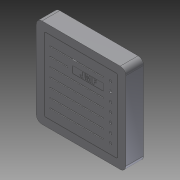
# Autodesk Inventor part: readerCase
Saved by Autodesk Inventor 2012 (Build 160160000, 160)
## iProperties
Created: 2013-12-15
Part Number: readerCase
Material: Default
Document SubType Name: Modeling
Designer: joe_000
Density: 1 g/cm^3
Author: joe_000
Autodesk Inventor part; units mm, degrees
ref_plane "YZ Plane" through (0, 0, 0) normal (1, 0, 0) x (0, 1, 0)
ref_plane "XZ Plane" through (0, 0, 0) normal (0, 1, 0) x (-1, 0, 0)
sketch "Sketch1" plane through (0, 0, 0) normal (0, 0, 1) x (1, 0, 0)
  line L0 (7.9375, 0) -> (119.0625, 0)
  line L1 (127, 7.9375) -> (127, 119.0625)
  line L2 (119.0625, 127) -> (7.9375, 127)
  line L3 (0, 119.0625) -> (0, 7.9375)
  arc A0 (119.0625, 0) -> (127, 7.9375) centre (119.0625, 7.9375) ccw
  arc A1 (127, 119.0625) -> (119.0625, 127) centre (119.0625, 119.0625) ccw
  arc A2 (7.9375, 127) -> (0, 119.0625) centre (7.9375, 119.0625) ccw
  arc A3 (0, 7.9375) -> (7.9375, 0) centre (7.9375, 7.9375) ccw
  point P0 (0, 0)
  point P1 (127, 0)
  point P2 (0, 127)
  dimension "d0" = 127
  dimension "d1" = 127
  dimension "d2" = 7.9375
  constraints: 8 end point, 8 point on circle, 8 tangent, 6 point on line, 4 centre point, 3 equal radius, 2 parallel, 1 horizontal, 1 perpendicular
  measures "d0" distance of point (0, 0) point (127, 0)
  measures "d1" distance of point (0, 127) point (0, 0)
  measures "d2" radius of A0
extrude "Extrusion1" add sketch "Sketch1" along normal blind 25.4
sketch "Sketch2" plane through (0, 0, 0) normal (0, 0, -1) x (-1, 0, 0)
  line L0 (-119.0625, 0) -> (-7.9375, 0) projected
  line L1 (0, 7.9375) -> (0, 119.0625) projected
  line L2 (-7.9375, 127) -> (-119.0625, 127) projected
  line L3 (-127, 119.0625) -> (-127, 7.9375) projected
  arc A0 (-127, 7.9375) -> (-119.0625, 0) centre (-119.0625, 7.9375) ccw projected
  line L4 (-119.0625, 125.4125) -> (-7.9375, 125.4125)
  line L5 (-1.5875, 119.0625) -> (-1.5875, 7.9375)
  line L6 (-7.9375, 1.5875) -> (-119.0625, 1.5875)
  line L7 (-125.4125, 7.9375) -> (-125.4125, 119.0625)
  arc A1 (-125.4125, 7.9375) -> (-119.0625, 1.5875) centre (-119.0625, 7.9375) ccw
  arc A2 (-119.0625, 125.4125) -> (-125.4125, 119.0625) centre (-119.0625, 119.0625) ccw
  arc A3 (-1.5875, 119.0625) -> (-7.9375, 125.4125) centre (-7.9375, 119.0625) ccw
  arc A4 (-7.9375, 1.5875) -> (-1.5875, 7.9375) centre (-7.9375, 7.9375) ccw
  point P0 (0, 0)
  dimension "d6" = 1.5875
  dimension "d7" = 1.5875
  dimension "d8" = 1.5875
  dimension "d9" = 1.5875
  dimension "d10" = 1.5875
  constraints: 8 end point, 8 point on circle, 8 tangent, 4 centre point, 3 equal radius, 2 parallel, 1 horizontal, 1 perpendicular
  measures "d6" distance between parallel lines of L3 L7
  measures "d7" distance between parallel lines of L2 L4
  measures "d8" distance between parallel lines of L1 L5
  measures "d9" distance between parallel lines of L0 L6
  measures "d10" radial gap between concentric circles of A0 A1
extrude "Extrusion2" cut sketch "Sketch2" against normal blind 23.8125
sketch "Sketch3" plane through (0, 0, 25.4) normal (0, 0, 1) x (1, 0, 0)
  line L0 (7.9375, 127) -> (119.0625, 127) projected
  line L1 (0, 7.9375) -> (0, 119.0625) projected
  line L2 (13.208, 115.824) -> (113.792, 115.824)
  line L3 (115.824, 113.792) -> (115.824, 13.208)
  line L4 (113.792, 11.176) -> (13.208, 11.176)
  line L5 (11.176, 13.208) -> (11.176, 113.792)
  line L6 (13.208, 115.4271) -> (113.792, 115.4271)
  line L7 (115.4271, 113.792) -> (115.4271, 13.208)
  line L8 (113.792, 11.5729) -> (13.208, 11.5729)
  line L9 (11.5729, 13.208) -> (11.5729, 113.792)
  arc A0 (13.208, 115.824) -> (11.176, 113.792) centre (13.208, 113.792) ccw
  arc A1 (11.176, 13.208) -> (13.208, 11.176) centre (13.208, 13.208) ccw
  arc A2 (113.792, 11.176) -> (115.824, 13.208) centre (113.792, 13.208) ccw
  arc A3 (115.824, 113.792) -> (113.792, 115.824) centre (113.792, 113.792) ccw
  arc A4 (13.208, 115.4271) -> (11.5729, 113.792) centre (13.208, 113.792) ccw
  arc A5 (115.4271, 113.792) -> (113.792, 115.4271) centre (113.792, 113.792) ccw
  arc A6 (113.792, 11.5729) -> (115.4271, 13.208) centre (113.792, 13.208) ccw
  arc A7 (11.5729, 13.208) -> (13.208, 11.5729) centre (13.208, 13.208) ccw
  point P0 (0, 0)
  dimension "d15" = 104.648
  dimension "d16" = 104.648
  dimension "d17" = 0.3969
  dimension "d18" = 0.3969
  dimension "d19" = 0.3969
  dimension "d20" = 0.3969
  dimension "d21" = 0.3969
  dimension "d22" = 11.176
  dimension "d23" = 11.176
  dimension "d24" = 2.032
  constraints: 16 end point, 16 point on circle, 16 tangent, 8 centre point, 6 equal radius, 4 parallel, 2 horizontal, 2 perpendicular
  measures "d15" distance between parallel lines of L4 L2
  measures "d16" distance between parallel lines of L3 L5
  measures "d17" distance between parallel lines of L2 L6
  measures "d18" distance between parallel lines of L3 L7
  measures "d19" distance between parallel lines of L4 L8
  measures "d20" distance between parallel lines of L5 L9
  measures "d21" radial gap between concentric circles of A0 A4
  measures "d22" distance between parallel lines of L1 L5
  measures "d23" distance between parallel lines of L0 L2
  measures "d24" radius of A0
extrude "Extrusion3" cut sketch "Sketch3" against normal blind 0.7937
sketch "Sketch4" plane through (0, 0, 25.4) normal (0, 0, 1) x (1, 0, 0)
  line L0 (119.0625, 0) -> (7.9375, 0) projected
  line L1 (127, 119.0625) -> (127, 7.9375) projected
  line L2 (0, 7.9375) -> (0, 119.0625) projected
  line L3 (19.304, 26.035) -> (95.504, 26.035)
  line L4 (95.504, 26.035) -> (95.504, 24.765)
  line L5 (95.504, 24.765) -> (19.304, 24.765)
  line L6 (19.304, 24.765) -> (19.304, 26.035)
  line L7 (19.304, 38.735) -> (95.504, 38.735)
  line L8 (95.504, 38.735) -> (95.504, 37.465)
  line L9 (95.504, 37.465) -> (19.304, 37.465)
  line L10 (19.304, 37.465) -> (19.304, 38.735)
  line L11 (19.304, 51.435) -> (95.504, 51.435)
  line L12 (95.504, 51.435) -> (95.504, 50.165)
  line L13 (95.504, 50.165) -> (19.304, 50.165)
  line L14 (19.304, 50.165) -> (19.304, 51.435)
  line L15 (19.304, 64.135) -> (95.504, 64.135)
  line L16 (95.504, 64.135) -> (95.504, 62.865)
  line L17 (95.504, 62.865) -> (19.304, 62.865)
  line L18 (19.304, 62.865) -> (19.304, 64.135)
  line L19 (19.304, 76.835) -> (95.504, 76.835)
  line L20 (95.504, 76.835) -> (95.504, 75.565)
  line L21 (95.504, 75.565) -> (19.304, 75.565)
  line L22 (19.304, 75.565) -> (19.304, 76.835)
  line L23 (19.304, 102.235) -> (95.504, 102.235)
  line L24 (95.504, 102.235) -> (95.504, 100.965)
  line L25 (95.504, 100.965) -> (19.304, 100.965)
  line L26 (19.304, 100.965) -> (19.304, 102.235)
  line L27 (19.304, 89.535) -> (44.704, 89.535)
  line L28 (44.704, 89.535) -> (44.704, 88.265)
  line L29 (44.704, 88.265) -> (19.304, 88.265)
  line L30 (19.304, 88.265) -> (19.304, 89.535)
  point P0 (0, 0)
  dimension "d27" = 24.765
  dimension "d28" = 1.27
  dimension "d29" = 19.304
  dimension "d30" = 76.2
  dimension "d33" = 12.7
  dimension "d40" = 76.2
  dimension "d45" = 25.4
  dimension "d46" = 12.7
  constraints: 56 end point, 4 parallel, 2 collinear, 2 horizontal, 2 perpendicular, 2 vertical, 40 other
  measures "d27" distance between parallel lines of L0 L5
  measures "d28" distance of L5.end L3.start
  measures "d29" distance between parallel lines of L2 L6
  measures "d30" distance of L4.end L5.end
  measures "d33" distance of L3.start L10.end
  measures "d40" distance of L3.end L23.end
  measures "d45" distance of L27.start L27.end
  measures "d46" distance from line of L29 L22.start
extrude "Extrusion4" cut sketch "Sketch4" against normal blind 0.7937
sketch "Sketch6" plane through (0, 0, 25.4) normal (0, 0, 1) x (1, 0, 0)
  line L0 (119.0625, 0) -> (7.9375, 0) projected
  line L1 (127, 119.0625) -> (127, 7.9375) projected
  circle A0 centre (105.41, 25.4) radius 1.905
  circle A1 centre (105.41, 38.1) radius 1.905
  circle A2 centre (105.41, 50.8) radius 1.905
  circle A3 centre (105.41, 63.5) radius 1.905
  circle A4 centre (105.41, 76.2) radius 1.905
  circle A5 centre (105.41, 88.9) radius 1.905
  circle A6 centre (105.41, 101.6) radius 1.905
  point P0 (0, 0)
  dimension "d53" = 3.81
  dimension "d56" = 12.7
  dimension "d61" = 21.59
  dimension "d62" = 25.4
  constraints: 7 centre point, 1 vertical, 12 other
  measures "d53" diameter of A0
  measures "d56" distance of A0.centre A1.centre
  measures "d61" distance from line of L1 A0.centre
  measures "d62" distance from line of L0 A0.centre
extrude "Extrusion6" cut sketch "Sketch6" against normal blind 0.7937
sketch "Sketch7" plane through (0, 0, 25.4) normal (0, 0, 1) x (1, 0, 0)
  circle A0 centre (105.41, 88.9) radius 1.905 projected
  circle A1 centre (105.41, 88.9) radius 1.905
  point P0 (0, 0)
  constraints: 1 centre point, 1 coincident, 1 concentric
extrude "Extrusion7" cut sketch "Sketch7" against normal up to next
sketch "Sketch5" plane through (0, 0, 25.4) normal (0, 0, 1) x (1, 0, 0)
  line L0 (19.304, 100.965) -> (19.304, 102.235) projected
  line L1 (19.304, 102.235) -> (95.504, 102.235) projected
  line L2 (95.504, 100.965) -> (19.304, 100.965) projected
  line L3 (51.054, 102.235) -> (56.134, 102.235)
  line L4 (56.134, 102.235) -> (56.134, 100.965)
  line L5 (56.134, 100.965) -> (51.054, 100.965)
  line L6 (51.054, 100.965) -> (51.054, 102.235)
  point P0 (0, 0)
  dimension "d49" = 5.08
  dimension "d50" = 31.75
  constraints: 8 end point, 2 parallel, 2 point on line, 1 horizontal, 1 perpendicular
  measures "d49" distance of L3.start L3.end
  measures "d50" distance between parallel lines of L0 L6
extrude "Extrusion5" cut sketch "Sketch5" against normal up to next contours L6 L1 L4 L2
sketch "Sketch8" plane through (0, 0, 25.4) normal (0, 0, 1) x (1, 0, 0)
  line L0 (7.9375, 127) -> (119.0625, 127) projected
  line L1 (52.324, 93.98) -> (94.234, 93.98)
  line L2 (95.504, 92.71) -> (95.504, 85.344)
  line L3 (94.234, 84.074) -> (52.324, 84.074)
  line L4 (51.054, 85.344) -> (51.054, 92.71)
  arc A0 (52.324, 93.98) -> (51.054, 92.71) centre (52.324, 92.71) ccw
  arc A1 (51.054, 85.344) -> (52.324, 84.074) centre (52.324, 85.344) ccw
  arc A2 (95.504, 92.71) -> (94.234, 93.98) centre (94.234, 92.71) ccw
  arc A3 (94.234, 84.074) -> (95.504, 85.344) centre (94.234, 85.344) ccw
  line L5 (95.504, 102.235) -> (95.504, 100.965) projected
  point P0 (0, 0)
  dimension "d67" = 1.27
  dimension "d68" = 9.906
  dimension "d69" = 44.45
  dimension "d70" = 33.02
  constraints: 8 end point, 8 point on circle, 8 tangent, 4 centre point, 3 equal radius, 2 parallel, 1 collinear, 1 horizontal, 1 perpendicular
  measures "d67" radius of A0
  measures "d68" distance between parallel lines of L3 L1
  measures "d69" distance between parallel lines of L2 L4
  measures "d70" distance between parallel lines of L0 L1
extrude "Extrusion8" cut sketch "Sketch8" against normal blind 0.3969
sketch "Sketch9" plane through (0, 0, 25.4) normal (0, 0, 1) x (1, 0, 0)
  line L0 (52.324, 93.98) -> (94.234, 93.98) projected
  line L1 (51.054, 85.344) -> (51.054, 92.71) projected
  line L2 (61.214, 92.837) -> (85.344, 92.837) construction
  line L3 (85.344, 92.837) -> (85.344, 85.217) construction
  line L4 (85.344, 85.217) -> (61.214, 85.217) construction
  line L5 (61.214, 85.217) -> (61.214, 92.837) construction
  line L6 (65.1597, 92.837) -> (67.5212, 92.837)
  line L7 (67.5212, 92.837) -> (67.5212, 88.6933)
  spline S0 degree 2 poles (67.5212, 88.6933) (67.5212, 87.3952) (67.0592, 86.0311) (65.6584, 85.085) (64.573, 85.085) knots 0 0 0 1 2 3 3 3
  spline S1 degree 2 poles (64.573, 85.085) (63.4215, 85.085) (62.1527, 85.7084) (61.4634, 86.9111) (61.3973, 87.7912) knots 0 0 0 1 2 3 3 3
  line L8 (61.3973, 87.7912) -> (63.6489, 88.0993)
  spline S2 degree 2 poles (63.6489, 88.0993) (63.6562, 87.5932) (63.8176, 87.1092) (64.0156, 86.9552) knots 0 0 0 1 2 2 2
  spline S3 degree 2 poles (64.0156, 86.9552) (64.1476, 86.8598) (64.3969, 86.8598) knots 0 0 0 1 1 1
  spline S4 degree 2 poles (64.3969, 86.8598) (64.793, 86.8598) (65.1597, 87.4465) (65.1597, 88.1433) knots 0 0 0 1 2 2 2
  line L9 (65.1597, 88.1433) -> (65.1597, 92.837)
  line L10 (69.076, 92.837) -> (72.1783, 92.837)
  line L11 (72.1783, 92.837) -> (73.3664, 88.2019)
  line L12 (73.3664, 88.2019) -> (74.5472, 92.837)
  line L13 (74.5472, 92.837) -> (77.6421, 92.837)
  line L14 (77.6421, 92.837) -> (77.6421, 85.217)
  line L15 (77.6421, 85.217) -> (75.7133, 85.217)
  line L16 (75.7133, 85.217) -> (75.7133, 91.0328)
  line L17 (75.7133, 91.0328) -> (74.2318, 85.217)
  line L18 (74.2318, 85.217) -> (72.4863, 85.217)
  line L19 (72.4863, 85.217) -> (71.0049, 91.0328)
  line L20 (71.0049, 91.0328) -> (71.0049, 85.217)
  line L21 (71.0049, 85.217) -> (69.076, 85.217)
  line L22 (69.076, 85.217) -> (69.076, 92.837)
  line L23 (79.1676, 92.837) -> (84.9834, 92.837)
  line L24 (84.9834, 92.837) -> (84.9834, 91.2015)
  line L25 (84.9834, 91.2015) -> (81.5364, 91.2015)
  line L26 (81.5364, 91.2015) -> (81.5364, 89.8741)
  line L27 (81.5364, 89.8741) -> (84.4774, 89.8741)
  line L28 (84.4774, 89.8741) -> (84.4774, 88.3339)
  line L29 (84.4774, 88.3339) -> (81.5364, 88.3339)
  line L30 (81.5364, 88.3339) -> (81.5364, 85.217)
  line L31 (81.5364, 85.217) -> (79.1676, 85.217)
  line L32 (79.1676, 85.217) -> (79.1676, 92.837)
  point P0 (0, 0)
  dimension "d74" = 1.143
  dimension "d75" = 10.16
  dimension "d76" = 24.13
  constraints: 2 other
  measures "d74" distance between parallel lines of L0 L2
  measures "d75" distance between parallel lines of L1 L5
  measures "d76" distance between parallel lines of L3 L5
extrude "Extrusion9" cut sketch "Sketch9" against normal blind 0.7937
sketch "Sketch10" plane through (0, 0, 23.8125) normal (0, 0, -1) x (-1, 0, 0)
  line L0 (-1.5875, 7.9375) -> (-1.5875, 119.0625) projected
  line L1 (-33.7625, 118.1275) -> (-1.5875, 118.1275)
  line L2 (-1.5875, 118.1275) -> (-1.5875, 8.8725)
  line L3 (-1.5875, 8.8725) -> (-33.7625, 8.8725)
  line L4 (-33.7625, 8.8725) -> (-33.7625, 118.1275)
  line L5 (-119.0625, 0) -> (-7.9375, 0) projected
  point P0 (0, 0)
  dimension "d79" = 109.255
  dimension "d80" = 8.8725
  dimension "d81" = 32.175
  constraints: 8 end point, 2 parallel, 1 horizontal, 1 perpendicular, 1 point on line
  measures "d79" distance of L3.end L1.start
  measures "d80" distance between parallel lines of L5 L3
  measures "d81" distance between parallel lines of L2 L4
extrude "Extrusion10" add sketch "Sketch10" along normal blind 16.0875
ref_plane "Work Plane2" through (1.5875, 10.46, 23.8125) normal (0, -1, 0) x (1, 0, 0)
sketch "Sketch12" plane through (1.5875, 10.46, 23.8125) normal (0, -1, 0) x (1, 0, 0)
  line L0 (0, -18.5759) -> (32.175, -18.5759)
  line L1 (32.175, 0) -> (32.175, -18.5759)
  line L2 (0, -18.5759) -> (0, 0)
  line L3 (1.5875, -18.5759) -> (1.5875, -8.7762)
  line L4 (30.5875, -18.5759) -> (30.5875, -8.7762)
  arc A0 (16.0875, -8.7762) -> (1.5875, -8.7762) centre (8.8375, -8.7762) ccw
  arc A1 (30.5875, -8.7762) -> (16.0875, -8.7762) centre (23.3375, -8.7762) ccw
  point P0 (-1.5875, -23.8125)
  dimension "d85" = 7.25
  dimension "d86" = 7.25
  dimension "d87" = 1.5875
  dimension "d88" = 1.5875
  constraints: 10 end point, 4 point on circle, 2 centre point, 2 horizontal alignment, 2 parallel, 2 point on line
  measures "d85" radius of A0
  measures "d86" radius of A1
  measures "d87" distance between parallel lines of L3 L2
  measures "d88" distance between parallel lines of L1 L4
extrude "Extrusion11" cut sketch "Sketch12" against normal blind 106.08
sketch "Sketch13" plane through (0, 0, 23.8125) normal (0, 0, -1) x (-1, 0, 0)
  line L0 (-125.4125, 119.0625) -> (-125.4125, 7.9375) projected
  line L1 (-119.0625, 1.5875) -> (-7.9375, 1.5875) projected
  circle A0 centre (-112.7125, 14.2875) radius 3.5
  circle A1 centre (-112.7125, 14.2875) radius 1.5
  circle A2 centre (-74.6125, 14.2875) radius 3.5
  circle A3 centre (-74.6125, 14.2875) radius 1.5
  circle A4 centre (-112.7125, 96.8375) radius 3.5
  circle A5 centre (-112.7125, 96.8375) radius 1.5
  circle A6 centre (-74.6125, 96.8375) radius 3.5
  circle A7 centre (-74.6125, 96.8375) radius 1.5
  point P0 (0, 0)
  dimension "d92" = 7
  dimension "d93" = 3
  dimension "d96" = 38.1
  dimension "d99" = 82.55
  dimension "d104" = 12.7
  dimension "d105" = 12.7
  constraints: 8 centre point, 4 coincident, 1 horizontal, 1 vertical, 12 other
  measures "d92" diameter of A0
  measures "d93" diameter of A1
  measures "d96" distance of A0.centre A2.centre
  measures "d99" distance of A0.centre A4.centre
  measures "d104" distance from line of L1 A1.centre
  measures "d105" distance from line of L0 A0.centre
extrude "Extrusion12" add sketch "Sketch13" along normal blind 10.38
equation "\"d7\" = d6"
equation "\"d8\" = d6"
equation "\"d9\" = d6"
equation "\"d10\" = d6"
equation "\"d16\" = d15"
equation "\"d18\" = d17"
equation "\"d19\" = d17"
equation "\"d20\" = d17"
equation "\"d21\" = d17"
equation "\"d22\" = -0.5 * d15 + 0.5 * d0"
equation "\"d23\" = d22"
equation "\"d40\" = 6 * d33"
equation "\"d46\" = d33"
equation "\"d56\" = d33"
equation "\"d75\" = -0.5 * d76 + 0.5 * d69"
equation "\"d80\" = -0.5 * d79 + 0.5 * d0"
equation "\"d85\" = 0.5 * AABatteryDiameter"
equation "\"d86\" = 0.5 * AABatteryDiameter"
equation "\"d90\" = 2 * AABatteryLength + AABatteryLengthSpace"
equation "\"AABatteryLengthSpace\" = 5.08"
equation "\"AABatteryDiameter\" = 14.5"
equation "\"AABatteryLength\" = 50.5"
body "Solid1"
